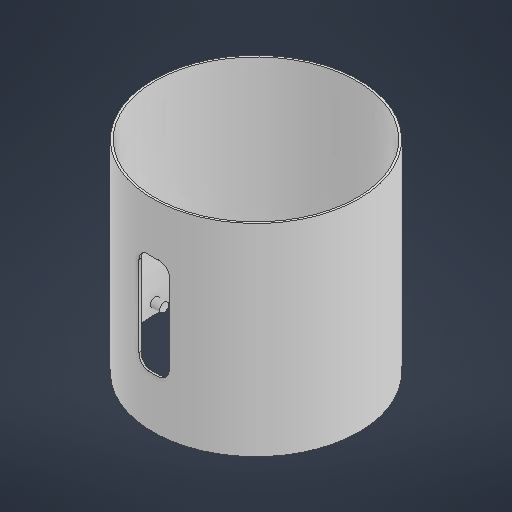
# Autodesk Inventor part: cover
Saved by Autodesk Inventor 2025.1 (Build 291241020, 241B)
## iProperties
Created: 2024-09-17
Part Number: cover
Material: Generic
Document SubType Name: Modeling
Designer: maxim
Density: 1 g/cm^3
Appearance: Default
Author: maxim
Autodesk Inventor part; units mm, degrees
ref_plane "XZ Plane" through (0, 0, 0) normal (0, 1, 0) x (-1, 0, 0)
ref_plane "XY Plane" through (0, 0, 0) normal (0, 0, 1) x (1, 0, 0)
sketch "Sketch1" plane through (0, 0, 0) normal (0, 1, 0) x (-1, 0, 0)
  circle A0 centre (0, 0) radius 100
  circle A1 centre (0, 0) radius 102
  dimension "d0" = 200
  dimension "d1" = 2
  constraints: 2 centre point, 1 coincident
  measures "d0" diameter of A0
  measures "d1" radial gap between concentric circles of A0 A1
extrude "Extrusion1" add sketch "Sketch1" along normal blind 200
sketch "Sketch2" plane through (0, 0, 0) normal (0, 0, 1) x (1, 0, 0)
  line L0 (-5, 50) -> (0, 50)
  line L1 (0, 150) -> (-5, 150)
  line L2 (-15, 140) -> (-15, 60)
  line L3 (102, 200) -> (-102, 200) projected
  line L4 (0, 200) -> (0, 0) construction
  line L5 (102, 0) -> (-102, 0) projected
  line L6 (-102, 200) -> (102, 0) construction
  line L7 (102, 200) -> (0, 100) construction
  line L8 (0, 100) -> (-15, 100) construction
  line L9 (5, 50) -> (0, 50)
  line L10 (0, 150) -> (5, 150)
  line L11 (15, 140) -> (15, 60)
  arc A0 (-5, 150) -> (-15, 140) centre (-5, 140) ccw
  arc A1 (15, 140) -> (5, 150) centre (5, 140) ccw
  arc A2 (-15, 60) -> (-5, 50) centre (-5, 60) ccw
  arc A3 (5, 50) -> (15, 60) centre (5, 60) ccw
  point P0 (-15, 50)
  point P1 (-15, 150)
  point P2 (15, 50)
  point P3 (15, 150)
  dimension "d4" = 15
  dimension "d5" = 100
  dimension "d9" = 10
  constraints: 20 end point, 10 point on line, 8 point on circle, 8 tangent, 4 centre point, 3 equal radius, 3 midpoint, 2 horizontal, 2 perpendicular, 2 symmetric about line, 1 parallel, 1 vertical
  measures "d4" distance between parallel lines of L4 L2
  measures "d5" distance of point (-15, 150) point (-15, 50)
  measures "d9" radius of A0
extrude "Extrusion2" cut sketch "Sketch2" along normal through all
ref_plane "Work Plane1" through (-101, 0, 0) normal (1, 0, 0) x (0, 1, 0)
sketch "Sketch3" plane through (-101, 0, 0) normal (1, 0, 0) x (0, 1, 0)
  circle A0 centre (10.5, 0) radius 4.5
  line L0 (0, 0) -> (200, 0) construction
  line L1 (200, -102) -> (200, 102) projected
  dimension "d11" = 9
  dimension "d12" = 10.5
  constraints: 2 end point, 1 centre point, 1 midpoint
  measures "d11" diameter of A0
  measures "d12" distance of L0.start A0.centre
extrude "Extrusion3" add sketch "Sketch3" along normal blind 10
pattern_circular "Circular Pattern1" count 2 over 360 about axis through (0, 0, 0) along (0, 1, 0) of "Extrusion3"
body "Solid1"
